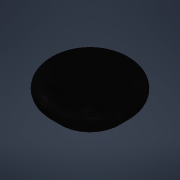
# Autodesk Inventor part: joystick
Saved by Autodesk Inventor 2022 (Build 260153000, 153)
## iProperties
Created: 2021-08-24
Part Number: joystick
Material: Gummi, Silikon
Document SubType Name: Modeling
Designer: Krillin
Density: 1.25 g/cm^3
Appearance: Eloxiert - Schwarz
Mass: 0.126932 g
Surface Area: 1.50137 cm^2
Volume: 0.101546 cm^3
Author: Krillin
Autodesk Inventor part; units mm, degrees
ref_plane "YZ Plane" through (0, 0, 0) normal (1, 0, 0) x (0, 1, 0)
ref_plane "XZ Plane" through (0, 0, 0) normal (0, 1, 0) x (-1, 0, 0)
ref_plane "XY Plane" through (0, 0, 0) normal (0, 0, 1) x (1, 0, 0)
sketch "Skizze1" plane through (0, 0, 0) normal (0, 1, 0) x (-1, 0, 0)
  circle A0 centre (0, 0) radius 4.039
  line L0 (0, 0) -> (1, 0)
  line L1 (1, 0) -> (1, 1)
  line L2 (1, 1) -> (0, 1)
  line L3 (0, 1) -> (0, 0)
  line L4 (1, 1) -> (-1, 1)
  line L5 (-1, 1) -> (-1, -1)
  line L6 (-1, -1) -> (1, -1)
  line L7 (1, -1) -> (1, 1)
  dimension "d10" = 1
  dimension "d11" = 1
  dimension "d12" = 2
  dimension "d13" = 2
  constraints: 16 end point, 4 parallel, 2 horizontal, 2 perpendicular, 1 centre point
  measures "d10" distance of L2.end L1.end
  measures "d11" distance of L1.end L0.end
  measures "d12" distance of L6.end L5.end
  measures "d13" distance of L5.end L4.end
extrude "Extrusion1" add sketch "Skizze1" along normal blind 3 contours A0 | L3 L2 L1 L0 | L0 L7 L6 L5 L4 L3
sketch "Skizze2" plane through (0, 3, 0) normal (0, 1, 0) x (1, 0, 0)
  circle A0 centre (0, 0) radius 2
  constraints: 1 centre point, 1 coincident
extrude "Extrusion2" add sketch "Skizze2" against normal blind 1
chamfer "Fase1" distance 1.4 angle 45 1 edges at (4.039, 0, 0)
sketch "Skizze3" plane through (0, 0, 0) normal (0, -1, 0) x (1, 0, 0)
  line L0 (0, 0) -> (1.1, 0)
  line L1 (1.1, 0) -> (1.1, -1.1)
  line L2 (1.1, -1.1) -> (0, -1.1)
  line L3 (0, -1.1) -> (0, 0)
  line L4 (1.1, -1.1) -> (-1.1, -1.1)
  line L5 (-1.1, -1.1) -> (-1.1, 1.1)
  line L6 (-1.1, 1.1) -> (1.1, 1.1)
  line L7 (1.1, 1.1) -> (1.1, -1.1)
  dimension "d14" = 1.1
  dimension "d15" = 1.1
  dimension "d16" = 2.2
  dimension "d17" = 2.2
  constraints: 16 end point, 4 parallel, 2 horizontal, 2 perpendicular
  measures "d14" distance of L1.end L2.end
  measures "d15" distance of L0.end L1.end
  measures "d16" distance of L5.end L6.end
  measures "d17" distance of L4.end L5.end
extrude "Extrusion3" cut sketch "Skizze3" against normal blind 2.7
fillet "Rundung4" radius 2 1 edges at (4.039, 3, 0)
fillet "Rundung5" radius 1 1 edges at (4.039, 1.4, 0)
